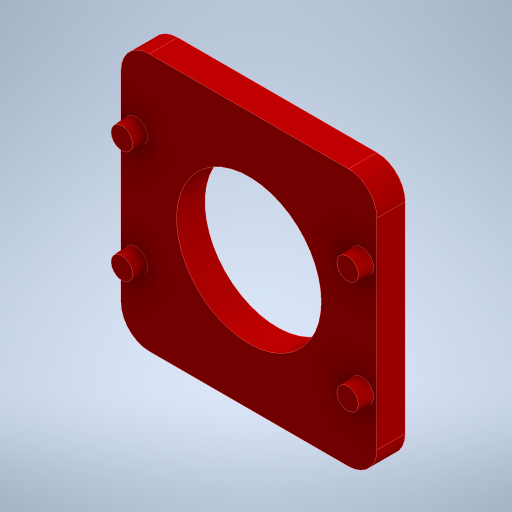
# Autodesk Inventor part: Filter Mount
Saved by Autodesk Inventor 2023.1 (Build 271208000, 208)
## iProperties
Created: 2022-11-16
Part Number: Filter Mount
Material: Generic
Document SubType Name: Modeling
Designer: xSibe
Density: 1 g/cm^3
Appearance: Plastic Dark Red
Author: xSibe
Autodesk Inventor part; units mm, degrees
ref_plane "YZ Plane" through (0, 0, 0) normal (1, 0, 0) x (0, 1, 0)
ref_plane "XZ Plane" through (0, 0, 0) normal (0, 1, 0) x (-1, 0, 0)
ref_plane "XY Plane" through (0, 0, 0) normal (0, 0, 1) x (1, 0, 0)
sketch "Sketch1" plane through (0, 0, 0) normal (0, 0, 1) x (1, 0, 0)
  line L0 (22.9, 0.025) -> (-22.9, 0.025) projected
  line L1 (22.9, 42.1) -> (22.9, 0.025) projected
  line L2 (22.9, 42.1) -> (17.05, 42.1) projected
  line L3 (17.05, 7.7) -> (17.05, 42.1) projected
  line L4 (-17.05, 7.7) -> (17.05, 7.7) projected
  line L5 (-17.05, 7.7) -> (-17.05, 42.1) projected
  line L6 (-17.05, 42.1) -> (-22.9, 42.1) projected
  line L7 (-22.9, 0.025) -> (-22.9, 42.1) projected
  circle A0 centre (19.9, 34.8) radius 2.0625 projected
  circle A1 centre (-19.9, 34.8) radius 2.0625 projected
  circle A2 centre (19.9, 15) radius 2.0625 projected
  circle A3 centre (-19.9, 15) radius 2.0625 projected
  circle A4 centre (10, 3.85) radius 1.5625 projected
  circle A5 centre (-10, 3.85) radius 1.5625 projected
  line L8 (-17.05, 7.7) -> (17.05, 7.7)
  line L9 (17.05, 7.7) -> (17.05, 42.1)
  line L10 (17.05, 42.1) -> (-17.05, 42.1)
  line L11 (-17.05, 42.1) -> (-17.05, 7.7)
  line L12 (-17.55, 47.6) -> (17.55, 47.6)
  line L13 (22.55, 42.6) -> (22.55, 7.2)
  line L14 (17.55, 2.2) -> (-17.55, 2.2)
  line L15 (-22.55, 7.2) -> (-22.55, 42.6)
  line L16 (-22.55, 24.9) -> (22.55, 24.9)
  circle A6 centre (0, 24.9) radius 12.75
  arc A7 (-17.55, 47.6) -> (-22.55, 42.6) centre (-17.55, 42.6) ccw
  arc A8 (22.55, 42.6) -> (17.55, 47.6) centre (17.55, 42.6) ccw
  arc A9 (17.55, 2.2) -> (22.55, 7.2) centre (17.55, 7.2) ccw
  arc A10 (-22.55, 7.2) -> (-17.55, 2.2) centre (-17.55, 7.2) ccw
  point P0 (0, 0)
  dimension "d0" = 5.5
  dimension "d1" = 25.5
  dimension "d2" = 5
  constraints: 18 end point, 8 point on circle, 8 tangent, 5 centre point, 4 parallel, 3 equal radius, 3 midpoint, 2 perpendicular, 1 horizontal, 3 other
  measures "d0" distance between parallel lines of L10 L12
  measures "d1" diameter of A6
  measures "d2" radius of A7
extrude "Extrusion1" add sketch "Sketch1" along normal mid plane 5 contours L13 L16 L3 L2 | L2 L10 L6 L15 A7 L12 A8 L13 | L6 L5 L16 L15 | L3 L16 A6 L5 L10 | L13 A9 L14 A10 L15 L16 L5 L4 L3 | L3 L4 L5 L16 A6 | A0 | A1 | A2 | A3 | A4 | A5
sketch "Sketch2" plane through (0, 0, 2.5) normal (0, 0, 1) x (1, 0, 0)
  line L0 (22.9, 0.025) -> (-22.9, 0.025) projected
  line L1 (22.9, 42.1) -> (22.9, 0.025) projected
  line L2 (22.9, 42.1) -> (17.05, 42.1) projected
  line L3 (17.05, 7.7) -> (17.05, 42.1) projected
  line L4 (-17.05, 7.7) -> (17.05, 7.7) projected
  line L5 (-17.05, 7.7) -> (-17.05, 42.1) projected
  line L6 (-17.05, 42.1) -> (-22.9, 42.1) projected
  line L7 (-22.9, 0.025) -> (-22.9, 42.1) projected
  circle A0 centre (19.9, 34.8) radius 2.0625 projected
  circle A1 centre (-19.9, 34.8) radius 2.0625 projected
  circle A2 centre (19.9, 15) radius 2.0625 projected
  circle A3 centre (-19.9, 15) radius 2.0625 projected
  circle A4 centre (10, 3.85) radius 1.5625 projected
  circle A5 centre (-10, 3.85) radius 1.5625 projected
  point P0 (0, 0)
extrude "Extrusion2" add sketch "Sketch2" along normal blind 2.5 contours A0 | A1 | A2 | A3
chamfer "Chamfer1" distance 2.5 angle 3.75 1 edges at (17.8375, 34.8, 5) measured on face at (21.7975, 35.6084, 4.1667)
chamfer "Chamfer2" distance 2.5 angle 3.75 1 edges at (17.8375, 15, 5) measured on face at (21.9358, 14.6692, 4.1667)
chamfer "Chamfer3" distance 2.5 angle 3.75 1 edges at (-21.9625, 34.8, 5) measured on face at (-18.0025, 35.6084, 4.1667)
chamfer "Chamfer4" distance 2.5 angle 3.75 1 edges at (-21.9625, 15, 5) measured on face at (-17.8642, 14.6692, 4.1667)
body "Solid1"
